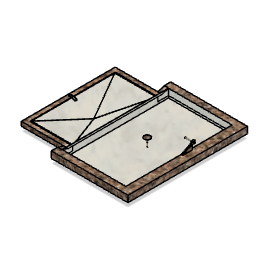
PoolProjectReal v4 (Autodesk Fusion 360 design; units mm, degrees)
Autodesk Fusion 360 part; units mm, degrees
note: some values were not read from the file. Set by a fixed rule: which face or edge a step refers to.
sketch "Sketch1" plane through (0, 0, 0) normal (0, 1, 0) x (1, 0, 0)
  line L0 (50, -100) -> (-50, -100)
  line L1 (-50, -100) -> (-50, 100)
  line L2 (-50, 100) -> (50, 100)
  line L3 (50, 100) -> (50, -100)
  line L4 (50, -100) -> (-50, 100) construction
  line L5 (-50, -100) -> (50, 100) construction
  dimension "d1" = 100
  dimension "d2" = 200
  constraint horizontal L0
  constraint perpendicular L0 L1
  constraint parallel L0 L2
  constraint parallel L1 L3
  constraint coincident L4 origin
  constraint coincident L5 origin
  measures "d1" distance of L1.end L2.end
  measures "d2" distance of L0.end L1.end
ref_plane "WorkPlane1" through (0, -20, 0) normal (0, 1, 0) x (1, 0, 0)
sketch "Sketch2" plane through (0, -20, 0) normal (0, 1, 0) x (1, 0, 0)
loft "Loft1" add profiles "Sketch1" section 1 section 2 point at (0, -20, 0) makes body 1
shell "Shell1" thickness 0.5 removed faces 1 at (16.6667, 0, 33.3333) on bodies 1
sketch "Sketch3" plane through (0, 0, 0) normal (0, 1, 0) x (-1, 0, 0)
  line L0 (48.6537, -97.4505) -> (-48.6537, -97.4505)
  line L1 (-48.6537, -97.4505) -> (-48.6537, 97.4505)
  line L2 (-48.6537, 97.4505) -> (48.6537, 97.4505)
  line L3 (48.6537, 97.4505) -> (48.6537, -97.4505)
  line L4 (-50, -100) -> (50, -100)
  line L5 (50, -100) -> (50, 100)
  line L6 (50, 100) -> (-50, 100)
  line L7 (-50, 100) -> (-50, -100)
  line L8 (50, -2.5) -> (57, -2.5)
  line L9 (57, -2.5) -> (57, 2.5)
  line L10 (57, 2.5) -> (50, 2.5)
  line L11 (50, 2.5) -> (50, -2.5)
  line L12 (50, -2.5) -> (48.6537, -2.5)
  line L13 (48.6537, -2.5) -> (48.6537, 2.5)
  line L14 (48.6537, 2.5) -> (50, 2.5)
  line L15 (50, 2.5) -> (50, -2.5)
  line L16 (48.6537, 2.5) -> (46.6537, 2.5)
  line L17 (46.6537, 2.5) -> (46.6537, -2.5)
  line L18 (46.6537, -2.5) -> (48.6537, -2.5)
  line L19 (48.6537, -2.5) -> (48.6537, 2.5)
  line L20 (-50, -125) -> (-200, -125)
  line L21 (-200, -125) -> (-200, 125)
  line L22 (-200, 125) -> (-50, 125)
  line L23 (-50, 125) -> (-50, -125)
  dimension "d5" = 7
  dimension "d6" = 5
  dimension "d7" = 97.5
  dimension "d9" = 97.5
  dimension "d14" = 2
  dimension "d33" = 150
  dimension "d34" = 250
  dimension "d35" = 25
  constraint horizontal L8
  constraint vertical L9
  constraint horizontal L10
  constraint vertical L11
  constraint coincident L5 L8.start
  constraint horizontal L12
  constraint vertical L13
  constraint horizontal L14
  constraint vertical L15
  constraint coincident L3 L13.end
  constraint collinear L10 L14
  constraint horizontal L16
  constraint vertical L17
  constraint horizontal L18
  constraint vertical L19
  constraint collinear L12 L18
  constraint horizontal L20
  constraint vertical L21
  constraint horizontal L22
  constraint vertical L23
  measures "d5" distance of L8.start L8.end
  measures "d6" distance of L8.start L10.end
  measures "d7" distance of L4.end L8
  measures "d9" distance of L5.end L10
  measures "d14" distance of L13.end L16.end
  measures "d33" distance of L20.start L20.end
  measures "d34" distance of L20.start L22.end
  measures "d35" distance of L6 L22.end
extrude "Extrude1" add sketch "Sketch3" against normal blind 3 separate body contours L5 L8 L9 L10 L11 L15 makes body 2
extrude "Extrude2" cut sketch "Sketch3" against normal blind 3 contours L3 L5 L11 L12 L13 L14 L15 L19 bodies 1
extrude "Extrude3" cut sketch "Sketch3" against normal blind 1.5 contours L3 L13 L16 L17 L18 L19 bodies 1
extrude "Extrude4" add 1 faces at (-50, -1, -0.8333) along direction (1, 0, 0) blind 3 on bodies 2 bodies 2 1
extrude "Extrude5" cut 1 faces at (-47, -1.8, 0.8333) along direction (1, 0, 0) blind 0.5 on bodies 2 bodies 2
extrude "Extrude6" add 1 faces at (-47, -1.8, 0.8333) along direction (1, 0, 0) blind 0.5 on bodies 2 bodies 2
sketch "Sketch4" plane through (-6.7109, -16.7771, 0) normal (0.371391, 0.928477, 0) x (0, 0, -1)
  line L0 (2.5, 45.1738) -> (2.5, 42.8542)
  line L1 (2.5, 42.8542) -> (-2.5, 42.8542)
  line L2 (-2.5, 42.8542) -> (-2.5, 45.1738)
  line L3 (-2.5, 45.1738) -> (-97.4505, 45.1738)
  line L4 (-97.4505, 45.1738) -> (-0.1431, -7.2278)
  line L5 (-0.1431, -7.2278) -> (0.1431, -7.2278)
  line L6 (0.1431, -7.2278) -> (97.4505, 45.1738)
  line L7 (97.4505, 45.1738) -> (2.5, 45.1738)
  line L8 (-2.5, 45.1738, 0) -> (-2.5, 43.1742, 0.7999)
  line L9 (-2.5, 43.1742, 0.7999) -> (-2.5, 42.8542, 0)
  point P0 (-2.5, 43.1742)
  constraint coincident L2.end L3.start
  constraint coincident L1.end L2.start
extrude "Extrude7" cut sketch "Sketch4" along normal blind 5 contours L2 L8 L9 in plane through (-6.7109, -16.7771, 2.5) normal (0, 0, -1) bodies 2
sketch "Sketch5" plane through (0, -3, 0) normal (0, -1, 0) x (1, 0, 0)
  line L0 (-46.5, 2.5) -> (-57, 2.5)
  line L1 (-57, 2.5) -> (-57, -2.5)
  line L2 (-57, -2.5) -> (-46.5, -2.5)
  line L3 (-46.5, -2.5) -> (-46.5, 2.5)
sketch "Sketch6" plane through (0, 0, -2.5) normal (0, 0, -1) x (-1, 0, 0)
  line L0 (57, 0) -> (50, 0)
  line L1 (50, 0) -> (46.5, -1.4)
  line L2 (46.5, -1.4) -> (46.5, -3)
  line L3 (46.5, -3) -> (57, -3)
  line L4 (57, -3) -> (57, 0)
  line L5 (46.5, -3) -> (41.2, -3)
  line L6 (41.2, -3) -> (46.5, -0.88)
  line L7 (48.6537, 0) -> (0, -19.4615)
  line L8 (46.5, -3) -> (46.5, -0.8615)
  constraint coincident L2.end L3.start
  constraint perpendicular L2 L5
  constraint parallel L1 L6
  constraint coincident L7 L8.end
  constraint perpendicular L3 L8
extrude "Extrude8" add sketch "Sketch6" against normal blind 5 contours L2 L5 L6 L8 bodies 2
sketch "Sketch7" plane through (0, 0, -2.5) normal (0, 0, -1) x (-1, 0, 0)
  line L0 (57, 0) -> (50, 0)
  line L1 (50, 0) -> (42.5, -3)
  line L2 (42.5, -3) -> (57, -3)
  line L3 (57, -3) -> (57, 0)
  line L4 (48.6537, 0) -> (0, -19.4615)
  line L5 (57, 0) -> (41.1537, -3)
  line L6 (41.1537, -3) -> (48.6537, 0)
  line L7 (57, 0) -> (48.6537, 0)
  constraint coincident L0.start L3.end
  constraint coincident L4 L5.end
  constraint coincident L4.start L6.end
  constraint parallel L4 L6
extrude "Extrude9" cut sketch "Sketch7" against normal blind 5 contours L0 L1 L5 L7 | L1 L4 L5 L6 L7 bodies 2
sketch "Sketch8" plane through (0, 0, -2.5) normal (0, 0, -1) x (-1, 0, 0)
  line L0 (57, 0) -> (43.7098, -2.5161)
  line L1 (43.7098, -2.5161) -> (42.5, -3)
  line L2 (42.5, -3) -> (57, -3)
  line L3 (57, -3) -> (57, 0)
  line L4 (50, 0) -> (50, -3)
  line L5 (50, -3) -> (42.5, -3)
  line L6 (50, 0) -> (42.5, -3)
  point P0 (50, 0)
  point P1 (50, 0)
  constraint coincident P1 P0
  constraint coincident L2 L4.end
  constraint coincident L1.end L2.start
extrude "Extrude10" add sketch "Sketch8" along normal blind 0.5 contours L0 L1 L2 L4 L5 L6 | L0 L4 L6 bodies 2
sketch "Sketch9" plane through (0, 0, 2.5) normal (0, 0, 1) x (1, 0, 0)
  line L0 (-43.7098, -2.5161) -> (-57, 0)
  line L1 (-57, 0) -> (-57, -3)
  line L2 (-57, -3) -> (-42.5, -3)
  line L3 (-42.5, -3) -> (-43.7098, -2.5161)
  line L4 (-50, 0) -> (-50, -3)
  line L5 (-50, -3) -> (-42.5, -3)
  line L6 (-50, 0) -> (-42.5, -3)
  point P0 (-50, 0)
  point P1 (-50, -3)
  point P2 (-50, -3)
  point P3 (-50, 0)
  constraint coincident P3 P0
  constraint coincident P2 P1
  constraint coincident L2.end L3.start
extrude "Extrude11" add sketch "Sketch9" along normal blind 0.5 contours L0 L2 L3 L4 L5 L6 | L0 L4 L6 bodies 2
extrude "Extrude12" add sketch "Sketch3" along normal blind 5 and the other way blind 15 separate body contours L7 L20 L21 L22 L23 makes body 3
sketch "Sketch10" plane through (0, 0, 0) normal (0, 0, 1) x (1, 0, 0)
  point P0 (125, 5)
sketch "Sketch11" plane through (0, 5, 0) normal (0, 1, 0) x (-1, 0, 0)
  line L0 (-50, 125) -> (-200, 125)
  line L1 (-200, 125) -> (-200, -125)
  line L2 (-200, -125) -> (-50, -125)
  line L3 (-50, -125) -> (-50, 125)
sketch "Sketch12" plane through (0, 5, 0) normal (0, 1, 0) x (-1, 0, 0)
  point P0 (-125, 0)
  point P1 (-125, 0)
  constraint coincident P0 P1
sketch "Sketch13" plane through (0, 5, 0) normal (0, 1, 0) x (-1, 0, 0)
  circle A0 centre (-125, 0) radius 7.5
  point P0 (-125, 0)
  dimension "d40" = 15
  constraint coincident P0 A0.centre
  measures "d40" diameter of A0
shell "Shell2" thickness 0.5 removed faces 1 at (150, 5, -41.6667) on bodies 3
ref_plane "WorkPlane2" through (125, -5, 0) normal (0, 1, 0) x (-1, 0, 0)
sketch "Sketch14" plane through (125, -5, 0) normal (0, 1, 0) x (1, 0, 0)
loft "Loft2" add profiles "Sketch13" section 1 section 2 point at (125, -5, 0) separate body makes body 4
sketch "Sketch15" plane through (0, -15, 0) normal (0, -1, 0) x (1, 0, 0)
  line L0 (200, 125) -> (50, 125)
  line L1 (50, 125) -> (50, -125)
  line L2 (50, -125) -> (200, -125)
  line L3 (200, -125) -> (200, 125)
  circle A0 centre (125, 0) radius 1
  point P0 (125, 0)
  dimension "d43" = 2
  constraint coincident P0 A0.centre
  measures "d43" diameter of A0
shell "Shell3" thickness 0.5 removed faces 1 at (123.0842, 5, 2.8099) on bodies 4
extrude "Extrude13" add sketch "Sketch15" against normal blind 10 contours A0 bodies 3 4
sketch "Sketch16" plane through (0, -14.5, 0) normal (0, 1, 0) x (-1, 0, 0)
  circle A0 centre (-125, 0) radius 1
  line L0 (-50.5, 124.5) -> (-199.5, 124.5)
  line L1 (-199.5, 124.5) -> (-199.5, -124.5)
  line L2 (-199.5, -124.5) -> (-50.5, -124.5)
  line L3 (-50.5, -124.5) -> (-50.5, 124.5)
  line L4 (-125, 0, 9.5) -> (-124, 0, 9.5)
  line L5 (-124, 0, 9.5) -> (-125, 0, 9.5)
  line L6 (-124, 0, 9.5) -> (-124, 0, 10.8)
  line L7 (-124, 0, 10.8) -> (-125, 0, 9.5)
  point P0 (-124, 0)
  point P1 (-124, 0)
  point P2 (-125, 0)
  point P3 (-125, 0)
  dimension "d48" = 1.3
  constraint coincident P1 P0
  constraint coincident P3 P2
  measures "d48" distance of P1 P0
revolve "Revolve1" add sketch "Sketch16" angle 360 about axis through (125, -15, 0) along (0, -1, 0) separate body contours L4 L5 L6 L7 in plane through (0, -14.5, 0) normal (0, 0, 1) makes body 5
sketch "Sketch17" plane through (0, 0, 0) normal (0, 1, 0) x (1, 0, 0)
  line L0 (-50, 100) -> (50, 100)
  line L1 (-50, -100) -> (-50, 100)
  line L2 (50, 100) -> (-50, 100)
  line L3 (50, 100) -> (50, 125)
  line L4 (50, 125) -> (200, 125)
  line L5 (200, 125) -> (200, -125)
  line L6 (200, -125) -> (50, -125)
  line L7 (50, -125) -> (50, -100)
  line L8 (50, -100) -> (-50, -100)
  line L9 (-60, -100) -> (-60, -110)
  line L10 (-60, -110) -> (40, -110)
  line L11 (40, -110) -> (40, -140)
  line L12 (40, -140) -> (220, -140)
  line L13 (220, -140) -> (220, 140)
  line L14 (220, 140) -> (40, 140)
  line L15 (40, 140) -> (40, 110)
  line L16 (40, 110) -> (-60, 110)
  line L17 (-60, 110) -> (-60, -100)
  point P0 (-50, -100)
  point P1 (-50, 100)
  point P2 (-50, 100)
  point P3 (50, 125)
  point P4 (200, 125)
  point P5 (200, -125)
  point P6 (50, -125)
  point P7 (50, -100)
  dimension "d49" = 10
  dimension "d50" = 10
  dimension "d51" = 15
  dimension "d52" = 10
  dimension "d53" = 10
  dimension "d54" = 10
  dimension "d55" = 15
  dimension "d56" = 20
  constraint coincident P0 L1.start
  constraint coincident P1 L0.start
  constraint coincident L0.end L2.start
  constraint coincident P2 P1
  constraint coincident P3 L3.end
  constraint coincident P4 L4.end
  constraint coincident P5 L5.end
  constraint coincident P6 L6.end
  constraint coincident P7 L7.end
  constraint vertical L9
  constraint perpendicular L9 L10
  constraint perpendicular L10 L11
  constraint perpendicular L5 L12
  constraint perpendicular L12 L13
  constraint perpendicular L5 L14
  constraint perpendicular L4 L15
  constraint perpendicular L5 L16
  constraint perpendicular L10 L17
  measures "d49" distance of L8 L10
  measures "d50" distance of L7 L11
  measures "d51" distance of L6 L12
  measures "d52" distance of L1 L17
  measures "d53" distance of L2 L16
  measures "d54" distance of L3 L15
  measures "d55" distance of L4 L14
  measures "d56" distance of L5 L13
extrude "Extrude14" add sketch "Sketch17" against normal blind 10 bodies 2 5 3
sketch "Sketch18" plane through (0, 0, 0) normal (0, 1, 0) x (-1, 0, 0)
  line L0 (50, -100) -> (50, -3)
  line L1 (-50, 100) -> (-50, -100)
  line L2 (50, 3) -> (50, 100)
  line L3 (-50, -100) -> (-50, -125)
  line L4 (-50, -125) -> (-200, -125)
  line L5 (-200, -125) -> (-200, 125)
  line L6 (-200, 125) -> (-50, 125)
  line L7 (-50, 125) -> (-50, 100)
  line L8 (60, -110) -> (60, 110)
  line L9 (60, 110) -> (-40, 110)
  line L10 (-40, 110) -> (-40, 140)
  line L11 (-40, 140) -> (-220, 140)
  line L12 (-220, 140) -> (-220, -140)
  line L13 (-220, -140) -> (-40, -140)
  line L14 (-40, -140) -> (-40, -110)
  line L15 (-40, -110) -> (60, -110)
  line L16 (50, 2.5) -> (50, -2.5)
  line L17 (50, -2.5) -> (48.6537, -2.5)
  line L18 (48.6537, -2.5) -> (48.6537, -97.4505)
  line L19 (48.6537, -97.4505) -> (-48.6537, -97.4505)
  line L20 (-48.6537, -97.4505) -> (-48.6537, 97.4505)
  line L21 (-48.6537, 97.4505) -> (48.6537, 97.4505)
  line L22 (48.6537, 97.4505) -> (48.6537, 2.5)
  line L23 (48.6537, 2.5) -> (50, 2.5)
  line L24 (-50.5, 124.5) -> (-50.5, -124.5)
  line L25 (-40, 110) -> (-50.5, 110)
  line L26 (-40, -110) -> (-50, -110)
  line L27 (-50, -125) -> (-40, -125)
  line L28 (-50, 125) -> (-40, 125)
  line L29 (50, 100) -> (-50, 100)
  line L30 (-50, -100) -> (50, -100)
  line L31 (50, -3) -> (50, -100)
  line L32 (50, -100) -> (-50, -100)
  line L33 (-50, 100) -> (50, 100)
  line L34 (50, 100) -> (50, 3)
  constraint coincident L9.end L10.start
  constraint coincident L24 L25.end
  constraint perpendicular L7 L25
  constraint coincident L14.end L15.start
  constraint coincident L3 L26.end
  constraint collinear L15 L26
  constraint coincident L3.end L4.start
  constraint midpoint L14 L27.end
  constraint coincident L6.end L7.start
  constraint midpoint L10 L28.end
sketch "Sketch19" plane through (0, 0, 0) normal (0, 1, 0) x (-1, 0, 0)
extrude "Extrude15" add sketch "Sketch18" along normal blind 5 separate body contours L7 L10 L25 L28 | L3 L14 L26 L27 makes body 6 at (43.3333, 0, 120) makes body 7 at (43.3333, 0, -115)
sketch "Sketch20" plane through (40, 0, 0) normal (-1, 0, 0) x (0, 0, 1)
  line L0 (-125, 0) -> (-110, 0)
  line L1 (-110, 0) -> (-110, 5)
  line L2 (-110, 5) -> (-125, 5)
  line L3 (-125, 5) -> (-125, 0)
  line L4 (-125, 5) -> (-110, 0)
  line L5 (110, 0) -> (125, 5)
  point P0 (110, 0)
  point P1 (125, 5)
  constraint coincident L2.end L3.start
  constraint coincident L0.end L1.start
  constraint coincident P0 L5.start
  constraint coincident P1 L5.end
split_face "SplitFace1" 1 faces at (40, 1.6667, 115) by curves path "Sketch20" along L5 on bodies 6
extrude "Extrude16" cut 1 faces at (40, 3.3333, 115) along direction (1, 0, 0) blind 10 on bodies 6 bodies 6
sketch "Sketch21" plane through (40, 0, 0) normal (-1, 0, 0) x (0, 0, 1)
  line L0 (-125, 0) -> (-110, 0)
  line L1 (-110, 0) -> (-110, 5)
  line L2 (-110, 5) -> (-125, 5)
  line L3 (-125, 5) -> (-125, 0)
  line L4 (-125, 5) -> (-110, 0)
  constraint coincident L2.end L3.start
  constraint coincident L0.end L1.start
extrude "Extrude17" cut sketch "Sketch21" against normal blind 10 contours L1 L2 L4 bodies 7
sketch "Sketch22" plane through (0, 0, 0) normal (0, 1, 0) x (-1, 0, 0)
  line L0 (50, -100) -> (50, -3)
  line L1 (-50, 100) -> (-50, -100)
  line L2 (50, 3) -> (50, 100)
  line L3 (-50, -100) -> (-50, -125)
  line L4 (-50, -125) -> (-200, -125)
  line L5 (-200, -125) -> (-200, 125)
  line L6 (-200, 125) -> (-50, 125)
  line L7 (-50, 125) -> (-50, 100)
  line L8 (60, -110) -> (60, 110)
  line L9 (60, 110) -> (-40, 110)
  line L10 (-40, 110) -> (-40, 140)
  line L11 (-40, 140) -> (-220, 140)
  line L12 (-220, 140) -> (-220, -140)
  line L13 (-220, -140) -> (-40, -140)
  line L14 (-40, -140) -> (-40, -110)
  line L15 (-40, -110) -> (60, -110)
  line L16 (50, 2.5) -> (50, -2.5)
  line L17 (50, -2.5) -> (48.6537, -2.5)
  line L18 (48.6537, -2.5) -> (48.6537, -97.4505)
  line L19 (48.6537, -97.4505) -> (-48.6537, -97.4505)
  line L20 (-48.6537, -97.4505) -> (-48.6537, 97.4505)
  line L21 (-48.6537, 97.4505) -> (48.6537, 97.4505)
  line L22 (48.6537, 97.4505) -> (48.6537, 2.5)
  line L23 (48.6537, 2.5) -> (50, 2.5)
  line L24 (-50, -125) -> (-40, -125)
  line L25 (-40, 125) -> (-50, 125)
  line L26 (50, 100) -> (-50, 100)
  line L27 (-50, -100) -> (50, -100)
  line L28 (50, -3) -> (50, -100)
  line L29 (50, -100) -> (-50, -100)
  line L30 (-50, 100) -> (50, 100)
  line L31 (50, 100) -> (50, 3)
  point P0 (-40, -125)
  point P1 (-40, 125)
  constraint coincident L3.end L4.start
  constraint coincident P0 L24.end
  constraint coincident P1 L25.start
  constraint coincident L6.end L7.start
split_face "SplitFace2" 1 faces at (213.3333, 0, 41.6667) by curves path "Sketch22" along L25 on bodies 2
extrude "Extrude18" add 1 faces at (153.3333, 0, 135) along direction (0, 1, 0) blind 5 on bodies 2 bodies 2 6
sketch "Sketch23" plane through (0, 0, -125) normal (0, 0, -1) x (-1, 0, 0)
  line L0 (-50, 0) -> (-40, 0)
  line L1 (-40, 0) -> (-40, 5)
  line L2 (-40, 5) -> (-50, 5)
  line L3 (-50, 5) -> (-50, 0)
  line L4 (-50, 0) -> (-40, 0)
  constraint coincident L0.start L3.end
  constraint coincident L0.end L1.start
extrude "Extrude19" add sketch "Sketch23" along normal blind 15 bodies 7 5 2
extrude "Extrude20" add 1 faces at (213.3333, 1.6667, 125) along direction (0, 0, -1) blind 265 on bodies 7 bodies 7
extrude "Extrude21" add 1 faces at (50, 3.3333, -130) along direction (1, 0, 0) blind 150 on bodies 7 bodies 7
sketch "Sketch24" plane through (0, 0, -110) normal (0, 0, -1) x (-1, 0, 0)
  line L0 (60, 0) -> (-40, 0)
  line L1 (-40, 0) -> (-40, -10)
  line L2 (-40, -10) -> (60, -10)
  line L3 (60, -10) -> (60, 0)
  line L4 (57, 0) -> (41.1537, -3)
  point P0 (57, 0)
  point P1 (41.1537, -3)
  constraint coincident P0 L4.start
  constraint coincident P1 L4.end
sketch "Sketch25" plane through (0, 0, 110) normal (0, 0, 1) x (1, 0, 0)
  line L0 (40, 0) -> (-60, 0)
  line L1 (-60, 0) -> (-60, -10)
  line L2 (-60, -10) -> (40, -10)
  line L3 (40, -10) -> (40, 0)
  line L4 (-46.6537, 0) -> (-41.1537, -3)
  point P0 (-46.6537, 0)
  point P1 (-41.1537, -3)
  constraint coincident P0 L4.start
  constraint coincident P1 L4.end
sketch "Sketch26" plane through (0, 0, 110) normal (0, 0, 1) x (1, 0, 0)
  line L0 (-50, 0) -> (-50, -1.3252)
  point P0 (-50, 0)
  point P1 (-50, -1.3252)
  constraint coincident P0 L0.start
  constraint coincident P1 L0.end
sketch "Sketch27" plane through (0, 0, 0) normal (0, 0, 1) x (1, 0, 0)
sketch "Sketch28" plane through (0, 0, 110) normal (0, 0, 1) x (1, 0, 0)
  line L0 (-57, 0) -> (-41.1537, -3)
  line L1 (-57, 0) -> (-50, -1.3252)
  line L2 (-50, 0) -> (-50, -1.3252)
  line L3 (-60, 0) -> (40, 0)
  line L4 (-57, 0) -> (-50, 0)
  line L5 (-57, 0) -> (-50, 0)
  line L6 (-50, 0) -> (-50, -1.3252)
  point P0 (-57, 0)
  point P1 (-50, -1.3252)
  point P2 (-50, 0)
  point P3 (-50, 0)
  point P4 (-57, 0)
  point P5 (-50, 0)
  point P6 (-50, -1.3252)
  constraint coincident P4 P0
  constraint coincident P1 L1.end
  constraint coincident P5 P3
extrude "Extrude22" cut sketch "Sketch3" against normal blind 1 contours L5 L8 L9 L10 L11 L15 bodies 7
sketch "Sketch29" plane through (0, 0, 0) normal (0, 1, 0) x (-1, 0, 0)
  line L0 (57, 2.5, 0) -> (41.1537, 2.5, -3)
  line L1 (41.1537, 2.5, -3) -> (48.6537, 2.5, 0)
  line L2 (48.6537, 2.5, 0) -> (41.1537, 2.5, -3)
  line L3 (48.6537, 2.5) -> (57, 2.5)
  point P0 (57, 2.5)
  point P1 (41.1537, 2.5)
  point P2 (48.6537, 2.5)
  point P3 (41.1537, 2.5)
  point P4 (48.6537, 2.5)
  point P5 (57, 2.5)
  constraint coincident P5 P0
  constraint coincident P3 P1
  constraint coincident P4 P2
extrude "Extrude23" cut sketch "Sketch29" against normal blind 5 contours L0 L1 L2 L3 in plane through (0, 0, 2.5) normal (0, 0, 1) bodies 7
sketch "Sketch30" plane through (0, 5, 0) normal (0, 1, 0) x (-1, 0, 0)
  line L0 (-50.5, 124.5) -> (-50.5, -124.5)
  line L1 (-50.5, -124.5) -> (-199.5, -124.5)
  line L2 (-199.5, -124.5) -> (-199.5, 124.5)
  line L3 (-199.5, 124.5) -> (-50.5, 124.5)
  line L4 (-50, -125) -> (-50, 125)
  line L5 (-50, 125) -> (-40, 125)
  line L6 (-40, 125) -> (-40, 140)
  line L7 (-40, 140) -> (-220, 140)
  line L8 (-220, 140) -> (-220, -140)
  line L9 (-220, -140) -> (-40, -140)
  line L10 (-40, -140) -> (-40, -125)
  line L11 (-40, -125) -> (-50, -125)
  line L12 (-199.5, -10.1081) -> (-203.5, -10.1081)
  line L13 (-203.5, -10.1081) -> (-203.5, -9.1081)
  line L14 (-203.5, -9.1081) -> (-199.5, -9.1081)
  line L15 (-199.5, -9.1081) -> (-199.5, -10.1081)
  line L16 (-199.5, -9.1081) -> (-203.5, -9.1081)
  line L17 (-203.5, -9.1081) -> (-203.5, -8.1081)
  line L18 (-203.5, -8.1081) -> (-199.5, -8.1081)
  line L19 (-199.5, -8.1081) -> (-199.5, -9.1081)
  line L20 (-199.5, -8.1081) -> (-203.5, -8.1081)
  line L21 (-203.5, -8.1081) -> (-203.5, -7.1081)
  line L22 (-203.5, -7.1081) -> (-199.5, -7.1081)
  line L23 (-199.5, -7.1081) -> (-199.5, -8.1081)
  line L24 (-199.5, -7.1081) -> (-220, -7.1081) construction
  line L25 (-199.5, -10.1081) -> (-220, -10.1081) construction
  line L26 (-199.5, -4.1081) -> (-220, -4.1081) construction
  line L27 (-203.5, -4.1081) -> (-203.5, -5.1081)
  line L28 (-199.5, -5.1081) -> (-199.5, -4.1081)
  line L29 (-203.5, -5.1081) -> (-199.5, -5.1081)
  line L30 (-199.5, -6.1081) -> (-199.5, -5.1081)
  line L31 (-203.5, -6.1081) -> (-199.5, -6.1081)
  line L32 (-203.5, -5.1081) -> (-203.5, -6.1081)
  line L33 (-203.5, -6.1081) -> (-203.5, -7.1081)
  line L34 (-203.5, -7.1081) -> (-199.5, -7.1081)
  line L35 (-199.5, -7.1081) -> (-199.5, -6.1081)
  line L36 (-199.5, -10.1081) -> (-203.5, -10.1081)
  line L37 (-199.5, -11.1081) -> (-203.5, -11.1081)
  line L38 (-199.5, -11.1081) -> (-199.5, -10.1081)
  line L39 (-203.5, -10.1081) -> (-203.5, -11.1081)
  line L40 (-203.5, -11.1081) -> (-203.5, -12.1081)
  line L41 (-203.5, -12.1081) -> (-203.5, -13.1081)
  line L42 (-199.5, -13.1081) -> (-199.5, -12.1081)
  line L43 (-199.5, -12.1081) -> (-199.5, -11.1081)
  line L44 (-203.5, -12.1081) -> (-199.5, -12.1081)
  line L45 (-203.5, -13.1081) -> (-199.5, -13.1081)
  line L46 (-203.5, -14.1081) -> (-199.5, -14.1081)
  line L47 (-203.5, -15.1081) -> (-199.5, -15.1081)
  line L48 (-199.5, -14.1081) -> (-199.5, -15.1081)
  line L49 (-199.5, -13.1081) -> (-199.5, -14.1081)
  line L50 (-203.5, -14.1081) -> (-203.5, -13.1081)
  line L51 (-203.5, -15.1081) -> (-203.5, -14.1081)
  line L52 (-203.5, -16.1081) -> (-203.5, -15.1081)
  line L53 (-199.5, -15.1081) -> (-199.5, -16.1081)
  dimension "d77" = 4
  dimension "d78" = 1
  dimension "d79" = 4
  dimension "d80" = 1
  dimension "d81" = 4
  dimension "d82" = 1
  constraint horizontal L12
  constraint vertical L13
  constraint horizontal L14
  constraint vertical L15
  constraint coincident L2 L12.start
  constraint horizontal L16
  constraint vertical L17
  constraint horizontal L18
  constraint vertical L19
  constraint horizontal L20
  constraint vertical L21
  constraint horizontal L22
  constraint vertical L23
  constraint coincident L8 L24.end
  constraint perpendicular L8 L24
  constraint coincident L8 L25.end
  constraint perpendicular L8 L25
  constraint symmetric L12.start L24 L26.start
  constraint symmetric L12.end L24 L27.start
  constraint symmetric L13.end L24 L27.end
  constraint symmetric L14.end L24 L28.start
  constraint symmetric L17.end L24 L31.start
  constraint symmetric L18.end L24 L30.start
  constraint symmetric L21.end L24 L22.start
  constraint symmetric L22.end L24 L23.start
  constraint symmetric L24 L25.end L26.end
  constraint symmetric L12.start L25 L15.end
  constraint symmetric L12.end L25 L13.start
  constraint symmetric L13.end L25 L37.end
  constraint symmetric L14.end L25 L37.start
  constraint symmetric L17.end L25 L40.end
  constraint symmetric L18.end L25 L42.end
  constraint symmetric L21.end L25 L41.end
  constraint symmetric L22.end L25 L42.start
  constraint symmetric L25 L26.start L53.end
  constraint symmetric L25 L27.start L52.start
  constraint symmetric L25 L27.end L47.start
  constraint symmetric L25 L28.start L47.end
  constraint symmetric L25 L30.start L46.end
  constraint symmetric L25 L31.start L46.start
  constraint symmetric L25 L21.end L41.end
  constraint symmetric L25 L22.end L42.start
  measures "d77" distance of L12.start L12.end
  measures "d78" distance of L12.start L14.end
  measures "d79" distance of L14.end L13.end
  measures "d80" distance of L14.end L18.end
  measures "d81" distance of L18.end L17.end
  measures "d82" distance of L18.end L22.end
sketch "Sketch31" plane through (0, 5, 0) normal (0, 1, 0) x (-1, 0, 0)
  line L0 (-203.5, -16.1081) -> (-203.5, -15.1081)
  line L1 (-199.5, -16.1081) -> (-203.5, -16.1081)
  line L2 (-203.5, -4.1081) -> (-199.5, -4.1081)
  point P0 (-199.5, -16.1081)
  point P1 (-203.5, -16.1081)
  point P2 (-203.5, -4.1081)
  point P3 (-199.5, -4.1081)
  constraint coincident P0 L1.start
  constraint coincident P1 L0.start
  constraint coincident P2 L2.start
  constraint coincident P3 L2.end
extrude "Extrude24" add sketch "Sketch30" along normal blind 0.5 separate body contours L2 L29 L30 L31 L32 makes body 8
extrude "Extrude25" add sketch "Sketch30" along normal blind 1 contours L2 L22 L31 L33 L34 L35 bodies 8 7
extrude "Extrude26" add sketch "Sketch30" along normal blind 1.5 separate body contours L2 L18 L20 L21 L22 L23 L34 makes body 9
extrude "Extrude27" add sketch "Sketch30" along normal blind 2 contours L2 L14 L16 L17 L18 L19 L20 bodies 9 8
extrude "Extrude28" add sketch "Sketch30" along normal blind 2.5 separate body contours L2 L12 L13 L14 L15 L16 L36 makes body 10
extrude "Extrude29" add sketch "Sketch30" along normal blind 3 contours L2 L12 L36 L37 L38 L39 bodies 10 9
extrude "Extrude30" add sketch "Sketch30" along normal blind 3.5 separate body contours L2 L37 L40 L43 L44 makes body 11
sketch "Sketch32" plane through (0, 5, 0) normal (0, 1, 0) x (-1, 0, 0)
  line L0 (-220, 140) -> (-220, -140)
  line L1 (-199.5, -12.1081) -> (-220, -12.1081) construction
  point P0 (-199.5, -12.1081)
  constraint coincident P0 L1.start
  constraint coincident L0 L1.end
  constraint perpendicular L0 L1
sketch "Sketch33" plane through (0, 5, 0) normal (0, 1, 0) x (-1, 0, 0)
  line L0 (-203.5, -11.1081) -> (-203.5, -5.1081)
  line L1 (-203.5, -5.1081) -> (-199.5, -5.1081)
  line L2 (-199.5, -5.1081) -> (-199.5, 124.5)
  line L3 (-199.5, 124.5) -> (-50.5, 124.5)
  line L4 (-50.5, 124.5) -> (-50.5, -124.5)
  line L5 (-50.5, -124.5) -> (-199.5, -124.5)
  line L6 (-199.5, -124.5) -> (-199.5, -11.1081)
  line L7 (-199.5, -11.1081) -> (-203.5, -11.1081)
  line L8 (-50, -125) -> (-50, 125)
  line L9 (-50, 125) -> (-40, 125)
  line L10 (-40, 125) -> (-40, 140)
  line L11 (-40, 140) -> (-220, 140)
  line L12 (-220, 140) -> (-220, -140)
  line L13 (-220, -140) -> (-40, -140)
  line L14 (-40, -140) -> (-40, -125)
  line L15 (-40, -125) -> (-50, -125)
  line L16 (-203.5, -4.1081) -> (-203.5, -5.1081)
  line L17 (-199.5, -5.1081) -> (-199.5, -4.1081)
  line L18 (-203.5, -4.1081) -> (-199.5, -4.1081)
  line L19 (-203.5, -6.1081) -> (-199.5, -6.1081)
  line L20 (-203.5, -5.1081) -> (-203.5, -6.1081)
  line L21 (-199.5, -6.1081) -> (-199.5, -5.1081)
  line L22 (-203.5, -7.1081) -> (-199.5, -7.1081)
  line L23 (-203.5, -6.1081) -> (-203.5, -7.1081)
  line L24 (-199.5, -7.1081) -> (-199.5, -6.1081)
  line L25 (-199.5, -7.1081) -> (-199.5, -8.1081)
  line L26 (-199.5, -8.1081) -> (-199.5, -9.1081)
  line L27 (-199.5, -9.1081) -> (-199.5, -10.1081)
  line L28 (-203.5, -9.1081) -> (-199.5, -9.1081)
  line L29 (-199.5, -8.1081) -> (-203.5, -8.1081)
  line L30 (-199.5, -10.1081) -> (-203.5, -10.1081)
  line L31 (-203.5, -10.1081) -> (-203.5, -9.1081)
  line L32 (-203.5, -9.1081) -> (-203.5, -8.1081)
  line L33 (-203.5, -8.1081) -> (-203.5, -7.1081)
extrude "Extrude31" add sketch "Sketch30" along normal blind 4 contours L2 L41 L42 L44 L45 bodies 11 10
extrude "Extrude32" add sketch "Sketch30" along normal blind 4.5 separate body contours L2 L45 L46 L49 L50 makes body 12
extrude "Extrude33" add sketch "Sketch30" along normal blind 5 contours L2 L46 L47 L48 L51 bodies 12 11
sketch "Sketch34" plane through (0, 5, 0) normal (0, 1, 0) x (-1, 0, 0)
  line L0 (-220, 140) -> (-220, -140)
  line L1 (-199.5, -16.1081) -> (-220, -16.1081)
  line L2 (-203.5, -5.1081) -> (-203.5, -15.1081)
  line L3 (-203.5, -15.1081) -> (-203.5, -14.1081)
  line L4 (-203.5, -14.1081) -> (-203.5, -13.1081)
  line L5 (-203.5, -13.1081) -> (-203.5, -12.1081)
  line L6 (-203.5, -12.1081) -> (-203.5, -11.1081)
  line L7 (-203.5, -11.1081) -> (-203.5, -10.1081)
  line L8 (-203.5, -10.1081) -> (-203.5, -9.1081)
  line L9 (-203.5, -9.1081) -> (-203.5, -8.1081)
  line L10 (-203.5, -8.1081) -> (-203.5, -7.1081)
  line L11 (-203.5, -7.1081) -> (-203.5, -6.1081)
  line L12 (-203.5, -6.1081) -> (-203.5, -5.1081)
  line L13 (-203.5, -15.1081) -> (-199.5, -15.1081)
  line L14 (-199.5, -15.1081) -> (-199.5, -14.1081)
  line L15 (-199.5, -14.1081) -> (-203.5, -14.1081)
  line L16 (-203.5, -14.1081) -> (-203.5, -15.1081)
  line L17 (-203.5, -14.1081) -> (-199.5, -14.1081)
  line L18 (-199.5, -14.1081) -> (-199.5, -13.1081)
  line L19 (-199.5, -13.1081) -> (-203.5, -13.1081)
  line L20 (-203.5, -13.1081) -> (-203.5, -14.1081)
  line L21 (-199.5, -14.1081) -> (-203.5, -14.1081)
  line L22 (-199.5, -14.1081) -> (-203.5, -14.1081)
  line L23 (-203.5, -14.1081) -> (-199.5, -14.1081)
  line L24 (-199.5, -13.1081) -> (-203.5, -13.1081)
  line L25 (-203.5, -13.1081) -> (-199.5, -13.1081)
  line L26 (-199.5, -13.1081) -> (-203.5, -13.1081)
  line L27 (-199.5, -12.1081) -> (-203.5, -12.1081)
  line L28 (-199.5, -12.1081) -> (-203.5, -12.1081)
  line L29 (-203.5, -12.1081) -> (-199.5, -12.1081)
  line L30 (-199.5, -11.1081) -> (-203.5, -11.1081)
  line L31 (-199.5, -11.1081) -> (-203.5, -11.1081)
  line L32 (-203.5, -11.1081) -> (-199.5, -11.1081)
  line L33 (-199.5, -10.1081) -> (-203.5, -10.1081)
  line L34 (-199.5, -10.1081) -> (-203.5, -10.1081)
  line L35 (-203.5, -10.1081) -> (-199.5, -10.1081)
  line L36 (-199.5, -9.1081) -> (-203.5, -9.1081)
  line L37 (-199.5, -9.1081) -> (-203.5, -9.1081)
  line L38 (-203.5, -9.1081) -> (-199.5, -9.1081)
  line L39 (-199.5, -8.1081) -> (-203.5, -8.1081)
  line L40 (-199.5, -8.1081) -> (-203.5, -8.1081)
  line L41 (-203.5, -8.1081) -> (-199.5, -8.1081)
  line L42 (-199.5, -7.1081) -> (-203.5, -7.1081)
  line L43 (-199.5, -7.1081) -> (-203.5, -7.1081)
  line L44 (-203.5, -7.1081) -> (-199.5, -7.1081)
  line L45 (-199.5, -6.1081) -> (-203.5, -6.1081)
  line L46 (-203.5, -6.1081) -> (-199.5, -6.1081)
  line L47 (-199.5, -6.1081) -> (-203.5, -6.1081)
  line L48 (-199.5, -5.1081) -> (-203.5, -5.1081)
  line L49 (-203.5, -5.1081) -> (-199.5, -5.1081)
  line L50 (-199.5, -13.1081) -> (-203.5, -13.1081)
  line L51 (-203.5, -12.1081) -> (-203.5, -13.1081)
  line L52 (-203.5, -13.1081) -> (-199.5, -13.1081)
  line L53 (-199.5, -13.1081) -> (-199.5, -12.1081)
  line L54 (-199.5, -12.1081) -> (-203.5, -12.1081)
  line L55 (-203.5, -12.1081) -> (-199.5, -12.1081)
  line L56 (-199.5, -12.1081) -> (-199.5, -11.1081)
  line L57 (-199.5, -11.1081) -> (-203.5, -11.1081)
  line L58 (-203.5, -11.1081) -> (-203.5, -12.1081)
  line L59 (-199.5, -11.1081) -> (-199.5, -10.1081)
  line L60 (-199.5, -10.1081) -> (-203.5, -10.1081)
  line L61 (-203.5, -10.1081) -> (-203.5, -11.1081)
  line L62 (-203.5, -11.1081) -> (-199.5, -11.1081)
  line L63 (-199.5, -9.1081) -> (-203.5, -9.1081)
  line L64 (-203.5, -9.1081) -> (-203.5, -10.1081)
  line L65 (-203.5, -10.1081) -> (-199.5, -10.1081)
  line L66 (-199.5, -10.1081) -> (-199.5, -9.1081)
  line L67 (-199.5, -9.1081) -> (-199.5, -8.1081)
  line L68 (-199.5, -8.1081) -> (-203.5, -8.1081)
  line L69 (-203.5, -8.1081) -> (-203.5, -9.1081)
  line L70 (-203.5, -9.1081) -> (-199.5, -9.1081)
  line L71 (-203.5, -7.1081) -> (-203.5, -8.1081)
  line L72 (-203.5, -8.1081) -> (-199.5, -8.1081)
  line L73 (-199.5, -8.1081) -> (-199.5, -7.1081)
  line L74 (-199.5, -7.1081) -> (-203.5, -7.1081)
  line L75 (-203.5, -6.1081) -> (-203.5, -7.1081)
  line L76 (-203.5, -7.1081) -> (-199.5, -7.1081)
  line L77 (-199.5, -7.1081) -> (-199.5, -6.1081)
  line L78 (-199.5, -6.1081) -> (-203.5, -6.1081)
  line L79 (-203.5, -5.1081) -> (-203.5, -6.1081)
  line L80 (-203.5, -6.1081) -> (-199.5, -6.1081)
  line L81 (-199.5, -6.1081) -> (-199.5, -5.1081)
  line L82 (-199.5, -5.1081) -> (-203.5, -5.1081)
  line L83 (-203.5, -19.1081) -> (-199.5, -19.1081)
  line L84 (-199.5, -18.1081) -> (-203.5, -18.1081)
  line L85 (-203.5, -17.1081) -> (-199.5, -17.1081)
  line L86 (-199.5, -20.1081) -> (-203.5, -20.1081)
  line L87 (-199.5, -21.1081) -> (-203.5, -21.1081)
  line L88 (-203.5, -22.1081) -> (-199.5, -22.1081)
  line L89 (-199.5, -23.1081) -> (-203.5, -23.1081)
  line L90 (-203.5, -24.1081) -> (-199.5, -24.1081)
  line L91 (-203.5, -25.1081) -> (-199.5, -25.1081)
  line L92 (-199.5, -26.1081) -> (-203.5, -26.1081)
  line L93 (-203.5, -27.1081) -> (-199.5, -27.1081)
  line L94 (-203.5, -26.1081) -> (-203.5, -27.1081)
  line L95 (-199.5, -26.1081) -> (-199.5, -27.1081)
  line L96 (-199.5, -25.1081) -> (-199.5, -26.1081)
  line L97 (-203.5, -27.1081) -> (-203.5, -17.1081)
  line L98 (-199.5, -24.1081) -> (-199.5, -25.1081)
  line L99 (-199.5, -23.1081) -> (-199.5, -24.1081)
  line L100 (-199.5, -22.1081) -> (-199.5, -23.1081)
  line L101 (-199.5, -21.1081) -> (-199.5, -22.1081)
  line L102 (-199.5, -20.1081) -> (-199.5, -21.1081)
  line L103 (-199.5, -19.1081) -> (-199.5, -20.1081)
  line L104 (-199.5, -18.1081) -> (-199.5, -19.1081)
  line L105 (-199.5, -17.1081) -> (-199.5, -18.1081)
  line L106 (-199.5, -16.1081) -> (-199.5, -17.1081)
  line L107 (-203.5, -16.1081) -> (-203.5, -17.1081)
  line L108 (-203.5, -16.1081) -> (-203.5, -15.1081)
  line L109 (-199.5, -16.1081) -> (-199.5, -15.1081)
  point P0 (-199.5, -16.1081)
  point P1 (-203.5, -15.1081)
  point P2 (-203.5, -16.1081)
  constraint coincident P0 L1.start
  constraint coincident L0 L1.end
  constraint perpendicular L0 L1
  constraint symmetric L1 L2.start L93.start
  constraint symmetric L1 P1 L85.start
  constraint symmetric L1 L11.end L92.end
  constraint symmetric L1 L13.end L85.end
  constraint symmetric L1 L14.end L84.start
  constraint symmetric L1 L18.end L83.end
  constraint symmetric L1 L3.end L84.end
  constraint symmetric L1 L4.end L83.start
  constraint symmetric L1 L27.start L86.start
  constraint symmetric L1 L5.end L86.end
  constraint symmetric L1 L30.start L87.start
  constraint symmetric L1 L6.end L87.end
  constraint symmetric L1 L33.start L88.end
  constraint symmetric L1 L7.end L88.start
  constraint symmetric L1 L36.start L89.start
  constraint symmetric L1 L8.end L89.end
  constraint symmetric L1 L39.start L90.end
  constraint symmetric L1 L9.end L90.start
  constraint symmetric L1 L42.start L91.end
  constraint symmetric L1 L10.end L91.start
  constraint symmetric L1 L45.start L92.start
  constraint symmetric L1 L48.start L93.end
  constraint coincident P2 L107.start
  constraint coincident P1 L2.end
  constraint coincident L13.end L14.start
extrude "Extrude34" add sketch "Sketch34" along normal blind 6 separate body contours L1 L85 L106 L107 makes body 13
sketch "Sketch35" plane through (0, 5, 0) normal (0, 1, 0) x (-1, 0, 0)
  line L0 (-199.5, -16.1081) -> (-203.5, -16.1081)
  line L1 (-203.5, -16.1081) -> (-203.5, -15.1081)
  line L2 (-203.5, -15.1081) -> (-199.5, -16.1081)
  line L3 (-199.5, -15.1081) -> (-199.5, -16.1081)
  line L4 (-203.5, -15.1081) -> (-199.5, -15.1081)
  point P0 (-199.5, -16.1081)
  point P1 (-203.5, -16.1081)
  point P2 (-203.5, -15.1081)
  point P3 (-199.5, -15.1081)
  constraint coincident P0 L0.start
  constraint coincident P1 L0.end
  constraint coincident P2 L1.end
  constraint coincident P3 L3.start
extrude "Extrude35" add sketch "Sketch35" along normal blind 5.5 separate body contours L2 L3 L4 makes body 14
extrude "Extrude36" add sketch "Sketch34" along normal blind 5.5 contours L1 L13 L108 L109 bodies 14 12 13
extrude "Extrude37" add sketch "Sketch34" along normal blind 6.5 separate body contours L84 L85 L97 L105 makes body 15
extrude "Extrude38" add sketch "Sketch34" along normal blind 7 contours L83 L84 L97 L104 bodies 15 14
extrude "Extrude39" add sketch "Sketch34" along normal blind 7.5 separate body contours L83 L86 L97 L103 makes body 16
extrude "Extrude40" add sketch "Sketch34" along normal blind 8 contours L86 L87 L97 L102 bodies 16 15
extrude "Extrude41" add sketch "Sketch34" along normal blind 8.5 separate body contours L87 L88 L97 L101 makes body 17
extrude "Extrude42" add sketch "Sketch34" along normal blind 9 contours L88 L89 L97 L100 bodies 17 16
extrude "Extrude43" add sketch "Sketch34" along normal blind 9.5 separate body contours L89 L90 L97 L99 makes body 18
extrude "Extrude44" add sketch "Sketch34" along normal blind 10 contours L90 L91 L97 L98 bodies 18 17
extrude "Extrude45" add sketch "Sketch34" along normal blind 10.5 separate body contours L91 L92 L96 L97 makes body 19
extrude "Extrude46" add sketch "Sketch34" along normal blind 11 contours L92 L93 L94 L95 L97 bodies 19 18
sketch "Sketch36" plane through (203.5, 0, 0) normal (1, 0, 0) x (0, 0, -1)
  line L0 (5.1081, 5) -> (27.1081, 5)
  line L1 (27.1081, 5) -> (27.1081, 16)
  line L2 (27.1081, 16) -> (26.1081, 16)
  line L3 (26.1081, 16) -> (26.1081, 15.5)
  line L4 (26.1081, 15.5) -> (25.1081, 15.5)
  line L5 (25.1081, 15.5) -> (25.1081, 15)
  line L6 (25.1081, 15) -> (24.1081, 15)
  line L7 (24.1081, 15) -> (24.1081, 14.5)
  line L8 (24.1081, 14.5) -> (23.1081, 14.5)
  line L9 (23.1081, 14.5) -> (23.1081, 14)
  line L10 (23.1081, 14) -> (22.1081, 14)
  line L11 (22.1081, 14) -> (22.1081, 13.5)
  line L12 (22.1081, 13.5) -> (21.1081, 13.5)
  line L13 (21.1081, 13.5) -> (21.1081, 13)
  line L14 (21.1081, 13) -> (20.1081, 13)
  line L15 (20.1081, 13) -> (20.1081, 12.5)
  line L16 (20.1081, 12.5) -> (19.1081, 12.5)
  line L17 (19.1081, 12.5) -> (19.1081, 12)
  line L18 (19.1081, 12) -> (18.1081, 12)
  line L19 (18.1081, 12) -> (18.1081, 11.5)
  line L20 (18.1081, 11.5) -> (17.1081, 11.5)
  line L21 (17.1081, 11.5) -> (17.1081, 11)
  line L22 (17.1081, 11) -> (16.1081, 11)
  line L23 (16.1081, 11) -> (16.1081, 10.5)
  line L24 (16.1081, 10.5) -> (15.1081, 10.5)
  line L25 (15.1081, 10.5) -> (15.1081, 10)
  line L26 (15.1081, 10) -> (14.1081, 10)
  line L27 (14.1081, 10) -> (14.1081, 9.5)
  line L28 (14.1081, 9.5) -> (13.1081, 9.5)
  line L29 (13.1081, 9.5) -> (13.1081, 9)
  line L30 (13.1081, 9) -> (12.1081, 9)
  line L31 (12.1081, 9) -> (12.1081, 8.5)
  line L32 (12.1081, 8.5) -> (11.1081, 8.5)
  line L33 (11.1081, 8.5) -> (11.1081, 8)
  line L34 (11.1081, 8) -> (10.1081, 8)
  line L35 (10.1081, 8) -> (10.1081, 7.5)
  line L36 (10.1081, 7.5) -> (9.1081, 7.5)
  line L37 (9.1081, 7.5) -> (9.1081, 7)
  line L38 (9.1081, 7) -> (8.1081, 7)
  line L39 (8.1081, 7) -> (8.1081, 6.5)
  line L40 (8.1081, 6.5) -> (7.1081, 6.5)
  line L41 (7.1081, 6.5) -> (7.1081, 6)
  line L42 (7.1081, 6) -> (6.1081, 6)
  line L43 (6.1081, 6) -> (6.1081, 5.5)
  line L44 (6.1081, 5.5) -> (5.1081, 5.5)
  line L45 (5.1081, 5.5) -> (5.1081, 5)
  line L46 (27.1081, 16) -> (35.1081, 16)
  line L47 (35.1081, 16) -> (35.1081, 15.5)
  line L48 (35.1081, 15.5) -> (27.1081, 15.5)
  line L49 (27.1081, 15.5) -> (27.1081, 16)
  dimension "d131" = 8
  constraint horizontal L46
  constraint vertical L47
  constraint horizontal L48
  constraint vertical L49
  constraint coincident L1.end L2.start
  constraint collinear L4 L48
  measures "d131" distance of L1.end L46.end
extrude "Extrude47" add sketch "Sketch36" against normal blind 4 separate body contours L1 L46 L47 L48 L49 makes body 20
sketch "Sketch37" plane through (0, 16, 0) normal (0, 1, 0) x (-1, 0, 0)
  line L0 (-203.5, -27.1081) -> (-203.5, -35.1081)
  line L1 (-203.5, -35.1081) -> (-199.5, -35.1081)
  line L2 (-199.5, -35.1081) -> (-199.5, -27.1081)
  line L3 (-199.5, -27.1081) -> (-203.5, -27.1081)
  line L4 (-203.5, -27.1081) -> (-199.5, -27.1081)
  line L5 (-201.5, -35.1081) -> (-201.5, -27.1081) construction
  line L6 (-199.5, -31.1081) -> (-203.5, -31.1081) construction
  point P0 (-202.5, -28.1081)
  point P1 (-200.5, -28.1081)
  point P2 (-202.5, -34.1081)
  point P3 (-200.5, -34.1081)
  dimension "d134" = 1
  dimension "d135" = 1
  constraint midpoint L1 L5.start
  constraint midpoint L4 L5.end
  constraint symmetric P0 L5 P1
  constraint midpoint L2 L6.start
  constraint midpoint L0 L6.end
  constraint symmetric P0 L6 P2
  constraint symmetric P1 L6 P3
  measures "d134" distance of P0 L4
  measures "d135" distance of L0 P0
sketch "Sketch38" plane through (0, 16, 0) normal (0, 1, 0) x (-1, 0, 0)
  circle A0 centre (-202.5, -28.1081) radius 0.25
  point P0 (-202.5, -28.1081)
  dimension "d133" = 0.5
  constraint coincident P0 A0.centre
  measures "d133" diameter of A0
sketch "Sketch39" plane through (0, 16, 0) normal (0, 1, 0) x (-1, 0, 0)
  circle A0 centre (-200.5, -28.1081) radius 0.25
  circle A1 centre (-200.5, -34.1081) radius 0.25
  circle A2 centre (-202.5, -34.1081) radius 0.25
  point P0 (-200.5, -28.1081)
  point P1 (-200.5, -34.1081)
  point P2 (-202.5, -34.1081)
  dimension "d136" = 0.5
  dimension "d137" = 0.5
  dimension "d138" = 0.5
  constraint coincident P0 A0.centre
  constraint coincident P1 A1.centre
  constraint coincident P2 A2.centre
  measures "d136" diameter of A0
  measures "d137" diameter of A1
  measures "d138" diameter of A2
extrude "Extrude48" add sketch "Sketch39" sketch "Sketch38" along normal blind 4 and the other way blind 11 of sketch 2 bodies 20 19
ref_plane "WorkPlane3" through (201.5, 20, -31.1081) normal (0, 1, 0) x (-1, 0, 0)
sketch "Sketch40" plane through (201.5, 20, -31.1081) normal (0, 1, 0) x (1, 0, 0)
  line L0 (-2, -4) -> (2, -4)
  line L1 (2, -4) -> (2, 4)
  line L2 (2, 4) -> (-2, 4)
  line L3 (-2, 4) -> (-2, -4)
  point P0 (-2, -4)
  dimension "d144" = 4
  dimension "d145" = 8
  constraint horizontal L0
  constraint vertical L1
  constraint horizontal L2
  constraint vertical L3
  constraint coincident P0 L0.start
  measures "d144" distance of L1.end L2.end
  measures "d145" distance of L0.end L1.end
ref_plane "WorkPlane4" through (201.5, 23, -31.1081) normal (0, 1, 0) x (1, 0, 0)
sketch "Sketch41" plane through (201.5, 23, -31.1081) normal (0, 1, 0) x (1, 0, 0)
loft "Loft3" add profiles "Sketch40" section 1 section 2 point at (201.5, 23, -31.1081) separate body makes body 21
sketch "Sketch42" plane through (199.5, 0, 0) normal (-1, 0, 0) x (0, 0, 1)
  line L0 (-35.1081, 15.5) -> (-27.1081, 15.5)
  line L1 (-27.1081, 15.5) -> (-27.1081, 5)
  line L2 (-27.1081, 5) -> (-124.5, 5)
  line L3 (-124.5, 5) -> (-124.5, -14.5)
  line L4 (-124.5, -14.5) -> (124.5, -14.5)
  line L5 (124.5, -14.5) -> (124.5, 5)
  line L6 (124.5, 5) -> (-5.1081, 5)
  line L7 (-5.1081, 5) -> (-5.1081, 5.5)
  line L8 (-5.1081, 5.5) -> (-6.1081, 5.5)
  line L9 (-6.1081, 5.5) -> (-6.1081, 6)
  line L10 (-6.1081, 6) -> (-7.1081, 6)
  line L11 (-7.1081, 6) -> (-7.1081, 6.5)
  line L12 (-7.1081, 6.5) -> (-8.1081, 6.5)
  line L13 (-8.1081, 6.5) -> (-8.1081, 7)
  line L14 (-8.1081, 7) -> (-9.1081, 7)
  line L15 (-9.1081, 7) -> (-9.1081, 7.5)
  line L16 (-9.1081, 7.5) -> (-10.1081, 7.5)
  line L17 (-10.1081, 7.5) -> (-10.1081, 8)
  line L18 (-10.1081, 8) -> (-11.1081, 8)
  line L19 (-11.1081, 8) -> (-11.1081, 8.5)
  line L20 (-11.1081, 8.5) -> (-12.1081, 8.5)
  line L21 (-12.1081, 8.5) -> (-12.1081, 9)
  line L22 (-12.1081, 9) -> (-13.1081, 9)
  line L23 (-13.1081, 9) -> (-13.1081, 9.5)
  line L24 (-13.1081, 9.5) -> (-14.1081, 9.5)
  line L25 (-14.1081, 9.5) -> (-14.1081, 10)
  line L26 (-14.1081, 10) -> (-15.1081, 10)
  line L27 (-15.1081, 10) -> (-15.1081, 10.5)
  line L28 (-15.1081, 10.5) -> (-16.1081, 10.5)
  line L29 (-16.1081, 10.5) -> (-16.1081, 11)
  line L30 (-16.1081, 11) -> (-17.1081, 11)
  line L31 (-17.1081, 11) -> (-17.1081, 11.5)
  line L32 (-17.1081, 11.5) -> (-18.1081, 11.5)
  line L33 (-18.1081, 11.5) -> (-18.1081, 12)
  line L34 (-18.1081, 12) -> (-19.1081, 12)
  line L35 (-19.1081, 12) -> (-19.1081, 12.5)
  line L36 (-19.1081, 12.5) -> (-20.1081, 12.5)
  line L37 (-20.1081, 12.5) -> (-20.1081, 13)
  line L38 (-20.1081, 13) -> (-21.1081, 13)
  line L39 (-21.1081, 13) -> (-21.1081, 13.5)
  line L40 (-21.1081, 13.5) -> (-22.1081, 13.5)
  line L41 (-22.1081, 13.5) -> (-22.1081, 14)
  line L42 (-22.1081, 14) -> (-23.1081, 14)
  line L43 (-23.1081, 14) -> (-23.1081, 14.5)
  line L44 (-23.1081, 14.5) -> (-24.1081, 14.5)
  line L45 (-24.1081, 14.5) -> (-24.1081, 15)
  line L46 (-24.1081, 15) -> (-25.1081, 15)
  line L47 (-25.1081, 15) -> (-25.1081, 15.5)
  line L48 (-25.1081, 15.5) -> (-26.1081, 15.5)
  line L49 (-26.1081, 15.5) -> (-26.1081, 16)
  line L50 (-26.1081, 16) -> (-35.1081, 16)
  line L51 (-35.1081, 16) -> (-35.1081, 15.5)
  circle A0 centre (-31.1081, 18) radius 1.75
  line L52 (-35.1081, 16) -> (-27.1081, 16)
  point P0 (-35.1081, 20)
  dimension "d147" = 3.5
  dimension "d148" = 2
  dimension "d149" = 4
  measures "d147" diameter of A0
  measures "d148" distance of A0.centre L52
  measures "d149" horizontal distance of A0.centre P0
extrude "Extrude49" add sketch "Sketch42" along normal blind 4 separate body contours A0 makes body 22
sketch "Sketch43" plane through (0, 5, 0) normal (0, 1, 0) x (-1, 0, 0)
sketch "Sketch44" plane through (195.5, 0, 0) normal (-1, 0, 0) x (0, 0, 1)
  circle A0 centre (-31.1081, 18) radius 1.75
sketch "Sketch45" plane through (195.5, 0, 0) normal (-1, 0, 0) x (0, 0, 1)
  point P0 (-31.1081, 18)
sketch "Sketch46" plane through (195.5, 0, 0) normal (-1, 0, 0) x (0, 0, 1)
  point P0 (-31.1081, 18)
extrude "Extrude50" add sketch "Sketch44" along normal blind 3 bodies 22
sketch "Sketch47" plane through (0, 5, 0) normal (0, 1, 0) x (-1, 0, 0)
sketch "Sketch48" plane through (192.5, 0, 0) normal (-1, 0, 0) x (0, 0, 1)
  circle A0 centre (-31.1081, 18) radius 1.75
sketch "Sketch49" plane through (192.5, 0, 0) normal (-1, 0, 0) x (0, 0, 1)
sketch "Sketch50" plane through (0, 0, 0) normal (0, 0, 1) x (1, 0, 0)
sketch "Sketch51" plane through (192.5, 0, 0) normal (-1, 0, 0) x (0, 0, 1)
  circle A0 centre (-31.1081, 18) radius 1.75
extrude "Extrude51" add sketch "Sketch48" along normal blind 10 bodies 22
sketch "Sketch52" plane through (0, 5, 0) normal (0, 1, 0) x (-1, 0, 0)
sketch "Sketch53" plane through (0, 5, 0) normal (0, 1, 0) x (-1, 0, 0)
  circle A0 through (-191.7203, -29.9293, -19.5) (-194.3453, -28.4137, -19.5) (-194.3453, -31.4448, -19.5)
  dimension "d160" = 3.5
